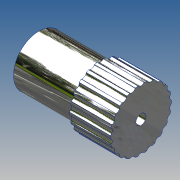
# Autodesk Inventor part: Nadelhalter_ra8846s
Saved by Autodesk Inventor 2021 (Build 250183000, 183)
## iProperties
Created: 2020-12-18
Part Number: Nadelhalter_ra8846s
Material: Aluminium 6061
Document SubType Name: Modeling
Designer: Ricardo
Density: 2.7 g/cm^3
Appearance: Aluminium - flach
Mass: 0.515134 g
Surface Area: 2.90722 cm^2
Volume: 0.19079 cm^3
Author: Sander
Revision Number: Rev00
Autodesk Inventor part; units mm, degrees
ref_plane "YZ-Ebene" through (0, 0, 0) normal (1, 0, 0) x (0, 1, 0)
ref_plane "XZ-Ebene" through (0, 0, 0) normal (0, 1, 0) x (-1, 0, 0)
ref_plane "XY-Ebene" through (0, 0, 0) normal (0, 0, 1) x (1, 0, 0)
sketch "Skizze1" plane through (0, 0, 0) normal (0, 0, 1) x (1, 0, 0)
  line L0 (-12, 0) -> (2, 0) projected
  line L1 (0, -0.6) -> (0, 3.6) projected
  line L2 (0, 3) -> (-4, 3)
  line L3 (-4, 3) -> (-4, 2.5)
  line L4 (-4, 2.5) -> (-10, 2.5)
  line L5 (-10, 2.5) -> (-10, 1.25)
  line L6 (-10, 1.25) -> (-3.5, 1.25)
  line L7 (-3.5, 1.25) -> (-3.5, 0.5)
  line L8 (-3.5, 0.5) -> (0, 0.5)
  point P0 (0, 0)
  dimension "d1" = 6
  dimension "d2" = 1
  dimension "d3" = 5
  dimension "d4" = 2.5
  dimension "d5" = 6.5
  dimension "d6" = 4
  dimension "d7" = 10
  constraints: 14 end point, 6 perpendicular, 2 point on line, 1 horizontal
  measures "d1" diameter of L2.start L0
  measures "d2" diameter of L8.end L0
  measures "d3" diameter of L4.end L0
  measures "d4" diameter of L5.end L0
  measures "d5" distance of L5.end L6.end
  measures "d6" distance of L2.start L2.end
  measures "d7" horizontal distance of L2.start L4.end
revolve "Umdrehung1" add sketch "Skizze1" angle 360 about axis through (-10, 0, 0) along (1, 0, 0)
sketch "Skizze2" plane through (0, 0, 0) normal (1, 0, 0) x (0, 0, -1)
  line L0 (0, -4.2) -> (0, 4.2) projected
  line L1 (4.33, 0) -> (-4.98, 0) projected
  circle A0 centre (-3.25, 0) radius 0.4
  dimension "d11" = 0.8
  dimension "d12" = 6.5
  constraints: 1 centre point, 1 point on line
  measures "d11" diameter of A0
  measures "d12" diameter of A0.centre L0
extrude "Extrusion1" cut sketch "Skizze2" against normal blind 4
pattern_circular "Runde Anordnung1" count 22 over 360 about axis through (-10, 0, 0) along (1, 0, 0) of "Extrusion1"
thread "Gewinde1" size "M3x0.5" class "6H" standard "ANSI Metric M Profile" length 7
